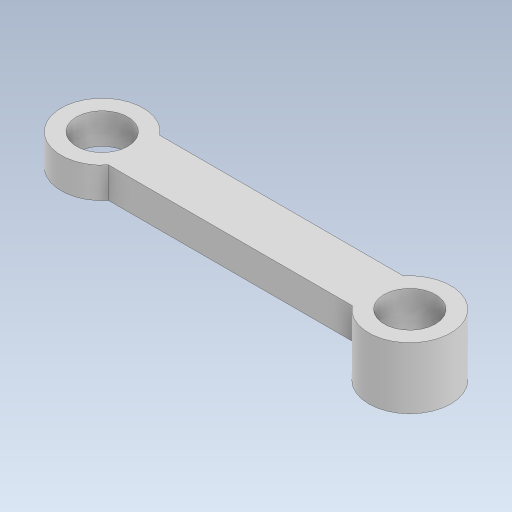
# Autodesk Inventor part: Arm Link
Saved by Autodesk Inventor 2023.5 (Build 275446000, 446)
## iProperties
Created: 2025-10-05
Part Number: Arm Link
Material: Generic
Document SubType Name: Modeling
Designer: Guntur
Density: 1 g/cm^3
Appearance: Default
Mass: 0.230385 g
Surface Area: 4.30131 cm^2
Volume: 0.230385 cm^3
Author: Guntur
## iProperties of the stored document Arm Link_3DPrint.ipt
Created: 2025-10-05
Part Number: Arm Link_3DPrint
Material: Generic
Document SubType Name: Modeling
Designer: Guntur
Density: 1 g/cm^3
Appearance: Default
Author: Guntur
Autodesk Inventor part; units mm, degrees
ref_plane "YZ Plane" through (0, 0, 0) normal (1, 0, 0) x (0, 1, 0)
ref_plane "XZ Plane" through (0, 0, 0) normal (0, 1, 0) x (-1, 0, 0)
ref_plane "XY Plane" through (0, 0, 0) normal (0, 0, 1) x (1, 0, 0)
sketch "Sketch1" plane through (0, 0, 0) normal (0, 1, 0) x (-1, 0, 0)
  circle A0 centre (0, 0) radius 2.5
  circle A1 centre (0, 0) radius 4
  circle A2 centre (-30, 0) radius 2.5
  circle A3 centre (-30, 0) radius 4
  line L0 (0, 2.5) -> (-30, 2.5)
  line L1 (-30, 2.5) -> (-30, -2.5)
  line L2 (-30, -2.5) -> (0, -2.5)
  line L3 (0, -2.5) -> (0, 2.5)
  point P0 (-3.4641, 2)
  point P1 (-26.5359, 2)
  point P2 (-26.5359, -2)
  point P3 (-3.4641, -2)
  point P4 (-27.2006, 2.8571)
  point P5 (-2.7994, 2.8571)
  point P6 (-2.7994, -2.8571)
  point P7 (-27.2006, -2.8571)
  point P8 (-26.8775, -2.5)
  point P9 (-3.1225, -2.5)
  point P10 (-3.1225, 2.5)
  point P11 (-26.8775, 2.5)
  dimension "d0" = 5
  dimension "d2" = 5
  dimension "d1" = 8
  dimension "d3" = 8
  dimension "d4" = 30
  constraints: 8 end point, 8 point on circle, 3 coincident, 2 centre point, 2 parallel, 2 vertical alignment, 1 horizontal, 1 perpendicular, 4 other
  measures "d1" diameter of A1
  measures "d3" diameter of A3
  measures "d4" distance of point (-30, 0) point (0, 0)
extrude "Extrusion1" add sketch "Sketch1" along normal blind 3 contours A0 L0 A1 L2 | A0 L2 A1 L0 | A1 L2 A3 L0 | L0 A2 L2 A3 | A3 L2 A2 L0
extrude "Extrusion2" add sketch "Sketch1" against normal blind 3 contours L0 A2 L2 A3 | A3 L2 A2 L0
body "Solid1"
